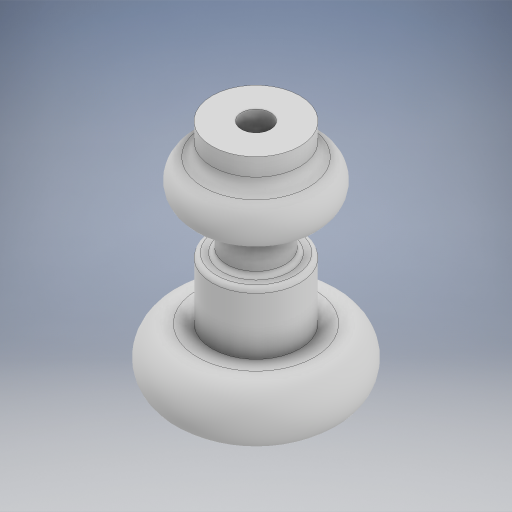
# Autodesk Inventor part: 1.2 pt 2
Saved by Autodesk Inventor 2024 (Build 280153000, 153)
## iProperties
Created: 2024-01-18
Part Number: 1.2 pt 2
Material: Generic
Document SubType Name: Modeling
Designer: Alex
Density: 1 g/cm^3
Appearance: Default
Author: Alex
Autodesk Inventor part; units mm, degrees
ref_plane "YZ Plane" through (0, 0, 0) normal (1, 0, 0) x (0, 1, 0)
ref_plane "XZ Plane" through (0, 0, 0) normal (0, 1, 0) x (-1, 0, 0)
ref_plane "XY Plane" through (0, 0, 0) normal (0, 0, 1) x (1, 0, 0)
sketch "Sketch2" plane through (0, 0, 0) normal (0, 0, 1) x (1, 0, 0)
  line L0 (0, 0) -> (0, 120)
  line L1 (0, 160) -> (10, 160) construction
  line L2 (30, 160) -> (30, 147.9129)
  line L3 (30, 0) -> (0, 0)
  line L4 (30, 0) -> (30, 40) construction
  line L5 (30, 0) -> (40, 0)
  arc A0 (30, 110) -> (36, 138.7477) centre (30, 125) ccw
  arc A1 (30, 147.9129) -> (36, 138.7477) centre (40, 147.9129) ccw
  arc A2 (30, 110) -> (20, 100) centre (30, 100) ccw
  line L6 (20, 100) -> (20, 85)
  line L7 (20, 0) -> (20, 85) construction
  line L8 (20, 0) -> (40, 0) construction
  arc A3 (20, 85) -> (23, 82) centre (23, 85) ccw construction
  line L9 (0, 82) -> (30, 82) construction
  arc A4 (30, 79) -> (27, 82) centre (27, 79) ccw construction
  arc A5 (20, 85) -> (23, 82) centre (23, 85) ccw
  arc A6 (30, 79) -> (27, 82) centre (27, 79) ccw
  line L10 (27, 82) -> (23, 82)
  line L11 (0, 0) -> (40, 0) construction
  line L12 (40, 0) -> (40, 20) construction
  line L13 (40, 20) -> (0, 20) construction
  line L14 (0, 20) -> (0, 0) construction
  arc A7 (40, 40) -> (40, 0) centre (40, 20) ccw construction
  line L15 (40, 40) -> (30, 40)
  line L16 (40, 0) -> (0, 0) construction
  arc A8 (40, 0) -> (40, 40) centre (40, 20) ccw
  line L17 (40, 0) -> (105, 0) construction
  line L18 (30, 40) -> (0, 40) construction
  line L19 (30, 40) -> (30, 125) construction
  arc A9 (27, 82) -> (30, 79) centre (27, 79) ccw construction
  line L20 (30, 79) -> (30, 40)
  line L21 (20, 85) -> (20, 0) construction
  arc A10 (23, 82) -> (20, 85) centre (23, 85) ccw construction
  line L22 (30, 147.9129) -> (30, 79) construction
  line L23 (0, 160) -> (10, 160) construction
  line L24 (10, 160) -> (10, 120)
  line L25 (10, 120) -> (0, 120)
  line L26 (0, 120) -> (0, 160) construction
  line L27 (10, 160) -> (30, 160)
  line L28 (0, 120) -> (0, 160) construction
  line L29 (0, 120) -> (0, 0)
  line L30 (40, 0) -> (155, 0) construction
  dimension "d0" = 160
  dimension "d1" = 30
  dimension "d2" = 125
  dimension "d3" = 90
  dimension "d4" = 30
  dimension "d5" = 20
  dimension "d6" = 20
  dimension "d7" = 85
  dimension "d8" = 90
  dimension "d9" = 6
  dimension "d10" = 85
  dimension "d11" = 30
  dimension "d12" = 6
  dimension "d13" = 40
  dimension "d14" = 20
  dimension "d15" = 10
  dimension "d16" = 40
  constraints: 62 end point, 22 point on circle, 18 tangent, 14 point on line, 12 perpendicular, 11 centre point, 10 collinear, 8 horizontal, 5 vertical, 4 coincident, 4 parallel
  measures "d0" distance of L0.start L1.start
  measures "d1" distance of L1.start L2.start
  measures "d2" distance of L3.start L19.end
  measures "d3" angle of L5 L4
  measures "d4" diameter of A0
  measures "d5" diameter of A1
  measures "d6" diameter of A2
  measures "d7" distance of L7.start L7.end
  measures "d8" angle of L8 L7
  measures "d9" diameter of A3
  measures "d10" distance from line of L3 A3.centre
  measures "d11" distance of L9.start L9.end
  measures "d12" diameter of A4
  measures "d13" distance of L13.end L12.end
  measures "d14" distance of L12.end L5.end
  measures "d15" distance of L24.end L0.end
  measures "d16" distance of L1.end L24.end
revolve "Revolution1" add sketch "Sketch2" angle 360 about axis through (0, 120, 0) along (0, 1, 0)
body "Solid1"
